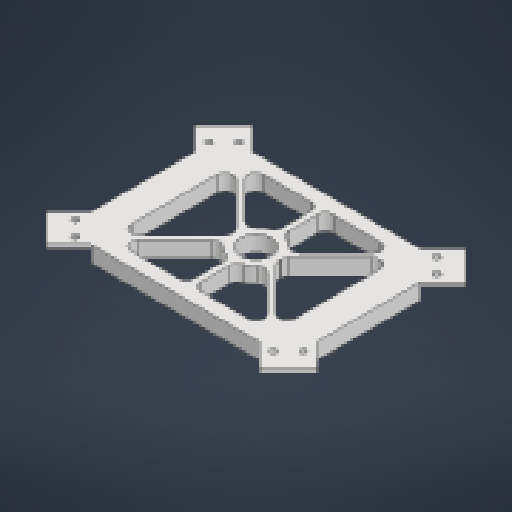
# Autodesk Inventor part: Base
Saved by Autodesk Inventor 2023 (Build 270158000, 158)
## iProperties
Created: 2023-01-21
Part Number: Base
Material: Generic
Document SubType Name: Modeling
Designer: Michael
Density: 1 g/cm^3
Appearance: Default
Author: Michael
Autodesk Inventor part; units mm, degrees
ref_plane "YZ Plane" through (0, 0, 0) normal (1, 0, 0) x (0, 1, 0)
ref_plane "XZ Plane" through (0, 0, 0) normal (0, 1, 0) x (-1, 0, 0)
ref_plane "XY Plane" through (0, 0, 0) normal (0, 0, 1) x (1, 0, 0)
sketch "Sketch1" plane through (0, 0, 0) normal (0, 1, 0) x (-1, 0, 0)
  line L0 (0, 0) -> (177.8, 0)
  line L1 (177.8, 0) -> (177.8, -127)
  line L2 (177.8, -127) -> (0, -127)
  line L3 (0, -127) -> (0, 0)
  line L4 (155.3506, 0) -> (177.8, -22.4519) projected
  line L5 (173.3121, 17.9595) -> (155.3506, 0) projected
  line L6 (195.7615, -4.4923) -> (173.3121, 17.9595) projected
  line L7 (177.8, -22.4519) -> (195.7615, -4.4923) projected
  line L8 (195.7615, -122.5077) -> (177.8, -104.5481) projected
  line L9 (173.3121, -144.9595) -> (195.7615, -122.5077) projected
  line L10 (155.3506, -127) -> (173.3121, -144.9595) projected
  line L11 (177.8, -104.5481) -> (155.3506, -127) projected
  line L12 (22.4494, 0) -> (4.4879, 17.9595) projected
  line L13 (0, -22.4519) -> (22.4494, 0) projected
  line L14 (4.4879, 17.9595) -> (-17.9615, -4.4923) projected
  line L15 (-17.9615, -4.4923) -> (0, -22.4519) projected
  line L16 (22.4494, -127) -> (0, -104.5481) projected
  line L17 (4.4879, -144.9595) -> (22.4494, -127) projected
  line L18 (0, -104.5481) -> (-17.9615, -122.5077) projected
  line L19 (-17.9615, -122.5077) -> (4.4879, -144.9595) projected
  circle A0 centre (178.6987, -10.7776) radius 2.4765
  circle A1 centre (167.025, 0.8974) radius 2.4765
  circle A2 centre (178.6987, -116.2224) radius 2.4765
  circle A3 centre (167.025, -127.8974) radius 2.4765
  circle A4 centre (10.775, -127.8974) radius 2.4765
  circle A5 centre (-0.8987, -116.2224) radius 2.4765
  circle A6 centre (-0.8987, -10.7776) radius 2.4765
  circle A7 centre (10.775, 0.8974) radius 2.4765
  dimension "d0" = 177.8
  dimension "d1" = 127
  constraints: 8 centre point, 8 end point, 2 parallel, 1 horizontal, 1 perpendicular, 16 other
  measures "d0" distance of L1.end L2.end
  measures "d1" distance of L0.end L1.end
extrude "Extrusion1" add sketch "Sketch1" along normal blind 12.7 contours L13 L3 A6 L0 A7 | L0 A7 L3 A6 L15 L14 L12 | L0 L4 L1 L11 L2 L16 L3 L13 | L5 L6 L7 L1 A0 L0 A1 | L0 A1 L1 A0 L4 | L16 L2 A4 L3 A5 | L3 A5 L2 A4 L17 L19 L18 | L8 L9 L10 L2 A3 L1 A2 | L1 A2 L2 A3 L11
sketch "Sketch6" plane through (0, 12.7, 0) normal (0, 1, 0) x (1, 0, 0)
  line L0 (-159.6708, 5.1549) -> (-18.3198, 5.1549)
  line L1 (-18.3198, 5.1549) -> (-18.3198, 121.9349)
  line L2 (-18.3198, 121.9349) -> (-159.6708, 121.9349)
  line L3 (-159.6708, 121.9349) -> (-159.6708, 5.1549)
  circle A0 centre (-88.9, 63.5) radius 12.2682
  line L4 (-24.5887, 14.5351) -> (-24.5887, 115.7894)
  line L5 (-24.5887, 115.7894) -> (-153.5245, 115.7894)
  line L6 (-153.5245, 115.7894) -> (-153.5245, 14.3771)
  line L7 (-153.5245, 112.7163) -> (-107.1207, 66.3124)
  line L8 (-153.5245, 112.7163) -> (-87.8995, 112.7163) construction
  line L9 (-150.4513, 115.7894) -> (-105.7361, 71.0742)
  line L10 (-153.5245, 14.3771) -> (-107.1207, 60.7809)
  line L11 (-150.4513, 11.3039) -> (-105.7651, 55.9901)
  line L12 (-24.5887, 112.7249) -> (-70.7001, 66.4653)
  line L13 (-27.4766, 115.7894) -> (-72.1058, 71.1763)
  line L14 (-24.4398, 14.3862) -> (-70.6864, 60.62)
  line L15 (-27.5134, 11.3039) -> (-72.0743, 55.8925)
  line L16 (-153.5245, 14.3771) -> (-107.1207, 60.7809)
  line L17 (-153.5245, 14.3771) -> (-153.5245, 63.5467)
  arc A1 (-70.6864, 60.62) -> (-70.7001, 66.4653) centre (-88.9, 63.5) ccw
  line L18 (-91.5188, 115.7894) -> (-91.519, 81.7746)
  line L19 (-86.6017, 115.7894) -> (-86.602, 81.8219)
  line L20 (-91.5188, 11.3039) -> (-91.519, 45.2251)
  line L21 (-86.6017, 11.3039) -> (-86.602, 45.1779)
  arc A2 (-86.602, 45.1779) -> (-72.0743, 55.8925) centre (-88.9, 63.5) ccw
  arc A3 (-72.1058, 71.1763) -> (-86.602, 81.8219) centre (-88.9, 63.5) ccw
  arc A4 (-91.519, 81.7746) -> (-105.7361, 71.0742) centre (-88.9, 63.5) ccw
  arc A5 (-107.1207, 66.3124) -> (-107.133, 60.7686) centre (-88.9, 63.5) ccw
  arc A6 (-105.7651, 55.9901) -> (-91.519, 45.2251) centre (-88.9, 63.5) ccw
  line L22 (-150.4513, 11.3039) -> (-91.5188, 11.3039)
  line L23 (-86.6017, 11.3039) -> (-27.5134, 11.3039)
  line L24 (-177.8, 104.5481) -> (-177.8, 22.4519) projected
  line L25 (0, 22.4519) -> (0, 104.5481) projected
  line L26 (0, 63.5) -> (-177.8, 63.5)
  line L27 (-22.4494, 127) -> (-155.3506, 127) projected
  line L28 (-88.9, 127) -> (-88.9, 0)
  point P0 (-203.2, 129.9481)
  point P1 (-203.2, 22.4519)
  point P2 (-180.7506, 0)
  point P3 (-22.4494, 0)
  point P4 (-25.3935, 140.9804)
  point P5 (-107.133, 60.7686)
  point P6 (-21.7778, 137.0134)
  point P7 (-177.8, 127)
  point P8 (-177.8, 0)
  dimension "d38" = 141.351
  dimension "d39" = 116.7799
  dimension "d42" = 24.5364
  dimension "d43" = 6.1463
  dimension "d45" = 45
  dimension "d46" = 45
  dimension "d47" = 3.0732
  dimension "d48" = 3.0732
  dimension "d54" = 4.917
  constraints: 60 end point, 12 point on circle, 9 point on line, 7 centre point, 5 parallel, 3 midpoint, 3 perpendicular, 2 collinear, 2 horizontal, 1 equal length, 1 vertical
  measures "d38" distance of L2.end L1.end
  measures "d39" distance of L1.end L0.end
  measures "d42" diameter of A0
  measures "d43" distance between parallel lines of L3 L6
  measures "d45" angle of L7 L8
  measures "d46" angle of L5 L9
  measures "d47" distance of L5.end L7.start
  measures "d48" distance of L9.start L5.end
  measures "d54" distance between parallel lines of L19 L18
extrude "Extrusion8" cut sketch "Sketch6" against normal blind 19.05 contours L28 L26 A0 | A0 L26 L28 | L26 A5 L10 L6 | L6 L7 A5 L26 | A0 L28 L26 | L26 L28 A0 | L26 A1 L12 L4 | L4 L14 A1 L26 | L5 L13 A3 L19 | L18 A4 L9 L5 | L11 A6 L20 L22 | L23 L21 A2 L15
fillet "Fillet1" radius 6.35 24 edges at (-70.7001, 6.35, -66.4653) (-70.6864, 6.35, -60.62) (-24.5887, 6.35, -14.5351) (-27.5134, 6.35, -11.3039) (-86.6017, 6.35, -11.3039) (-86.602, 6.35, -45.1779) (-72.0743, 6.35, -55.8925) (-86.6017, 6.35, -115.7894) (-86.602, 6.35, -81.8219) (-72.1058, 6.35, -71.1763) (-91.519, 6.35, -81.7746) (-105.7361, 6.35, -71.0742) (-150.4513, 6.35, -115.7894) (-91.5188, 6.35, -115.7894) (-153.5245, 6.35, -112.7163) (-107.1207, 6.35, -66.3124) (-107.133, 6.35, -60.7686) (-153.5245, 6.35, -14.3771) (-150.4513, 6.35, -11.3039) (-105.7651, 6.35, -55.9901) (-91.519, 6.35, -45.2251) (-91.5188, 6.35, -11.3039) (-27.4766, 6.35, -115.7894) (-24.5887, 6.35, -112.7249)
sketch "Sketch7" plane through (0, 0, 0) normal (0, -1, 0) x (1, 0, 0)
  arc A0 (-95.5736, -46.2868) -> (-102.0931, -50.5859) centre (-88.9, -63.5) ccw projected
  arc A1 (-111.1211, -50.6342) -> (-102.0931, -50.5859) centre (-106.631, -46.144) ccw projected
  line L0 (-111.1211, -50.6342) -> (-139.6112, -22.144) projected
  arc A2 (-135.1211, -11.3039) -> (-139.6112, -22.144) centre (-135.1211, -17.6539) ccw projected
  line L1 (-135.1211, -11.3039) -> (-97.8688, -11.3039) projected
  arc A3 (-91.5188, -17.6539) -> (-97.8688, -11.3039) centre (-97.8688, -17.6539) ccw projected
  line L2 (-91.5188, -17.6539) -> (-91.519, -40.3662) projected
  arc A4 (-95.5736, -46.2868) -> (-91.519, -40.3662) centre (-97.869, -40.3662) ccw projected
  circle A5 centre (-88.9, -63.5) radius 12.2682 projected
  line L3 (-153.5245, -97.386) -> (-153.5245, -29.7073) projected
  arc A6 (-142.6844, -25.2172) -> (-153.5245, -29.7073) centre (-147.1745, -29.7073) ccw projected
  line L4 (-142.6844, -25.2172) -> (-109.1944, -58.7071) projected
  arc A7 (-107.3351, -63.2748) -> (-109.1944, -58.7071) centre (-113.6846, -63.1972) ccw projected
  arc A8 (-107.3351, -63.2748) -> (-107.3341, -63.7937) centre (-88.9, -63.5) ccw projected
  arc A9 (-109.1932, -68.3849) -> (-107.3341, -63.7937) centre (-113.6833, -63.8948) ccw projected
  line L5 (-109.1932, -68.3849) -> (-142.6844, -101.8762) projected
  arc A10 (-153.5245, -97.386) -> (-142.6844, -101.8762) centre (-147.1745, -97.386) ccw projected
  line L6 (-24.5887, -29.8623) -> (-24.5887, -97.3598) projected
  arc A11 (-35.436, -101.8427) -> (-24.5887, -97.3598) centre (-30.9387, -97.3598) ccw projected
  line L7 (-35.436, -101.8427) -> (-68.6141, -68.558) projected
  arc A12 (-70.4651, -63.9278) -> (-68.6141, -68.558) centre (-64.1168, -64.0751) ccw projected
  arc A13 (-70.4651, -63.9278) -> (-70.4635, -63.1496) centre (-88.9, -63.5) ccw projected
  arc A14 (-68.6041, -58.5382) -> (-70.4635, -63.1496) centre (-64.1146, -63.029) ccw projected
  line L8 (-68.6041, -58.5382) -> (-35.4282, -25.3716) projected
  arc A15 (-24.5887, -29.8623) -> (-35.4282, -25.3716) centre (-30.9387, -29.8623) ccw projected
  line L9 (-42.8108, -115.7894) -> (-80.2518, -115.7894) projected
  arc A16 (-86.6018, -109.4395) -> (-80.2518, -115.7894) centre (-80.2518, -109.4394) ccw projected
  line L10 (-86.6018, -109.4395) -> (-86.6019, -86.7598) projected
  arc A17 (-82.4649, -80.8078) -> (-86.6019, -86.7598) centre (-80.2519, -86.7598) ccw projected
  arc A18 (-82.4649, -80.8078) -> (-75.7912, -76.505) centre (-88.9, -63.5) ccw projected
  arc A19 (-66.7939, -76.4863) -> (-75.7912, -76.505) centre (-71.2832, -80.9773) ccw projected
  line L11 (-66.7939, -76.4863) -> (-38.3215, -104.9485) projected
  arc A20 (-42.8108, -115.7894) -> (-38.3215, -104.9485) centre (-42.8108, -109.4394) ccw projected
  line L12 (-97.8688, -115.7894) -> (-135.1211, -115.7894) projected
  arc A21 (-139.6112, -104.9493) -> (-135.1211, -115.7894) centre (-135.1211, -109.4394) ccw projected
  line L13 (-139.6112, -104.9493) -> (-111.0747, -76.4128) projected
  arc A22 (-102.0585, -76.449) -> (-111.0747, -76.4128) centre (-106.5845, -80.9029) ccw projected
  arc A23 (-102.0585, -76.449) -> (-95.5735, -80.713) centre (-88.9, -63.5) ccw projected
  arc A24 (-91.519, -86.6335) -> (-95.5735, -80.713) centre (-97.869, -86.6336) ccw projected
  line L14 (-91.519, -86.6335) -> (-91.5188, -109.4394) projected
  arc A25 (-97.8688, -115.7894) -> (-91.5188, -109.4394) centre (-97.8688, -109.4394) ccw projected
  arc A26 (-75.7558, -50.5304) -> (-82.4649, -46.1919) centre (-88.9, -63.5) ccw projected
  arc A27 (-86.6019, -40.24) -> (-82.4649, -46.1919) centre (-80.2519, -40.24) ccw projected
  line L15 (-86.6019, -40.24) -> (-86.6018, -17.6539) projected
  arc A28 (-80.2518, -11.3039) -> (-86.6018, -17.6539) centre (-80.2518, -17.6539) ccw projected
  line L16 (-80.2518, -11.3039) -> (-42.8369, -11.3039) projected
  arc A29 (-38.3454, -22.1426) -> (-42.8369, -11.3039) centre (-42.8369, -17.6539) ccw projected
  line L17 (-38.3454, -22.1426) -> (-66.7442, -50.5591) projected
  arc A30 (-75.7558, -50.5304) -> (-66.7442, -50.5591) centre (-71.2358, -46.0704) ccw projected
  line L18 (-195.7615, -4.4923) -> (-173.3121, 17.9595) projected
  line L19 (-177.8, -22.4519) -> (-195.7615, -4.4923) projected
  line L20 (-177.8, -104.5481) -> (-177.8, -22.4519) projected
  line L21 (-195.7615, -122.5077) -> (-177.8, -104.5481) projected
  line L22 (-173.3121, -144.9595) -> (-195.7615, -122.5077) projected
  line L23 (-155.3506, -127) -> (-173.3121, -144.9595) projected
  line L24 (-22.4494, -127) -> (-155.3506, -127) projected
  line L25 (-4.4879, -144.9595) -> (-22.4494, -127) projected
  line L26 (17.9615, -122.5077) -> (-4.4879, -144.9595) projected
  line L27 (0, -104.5481) -> (17.9615, -122.5077) projected
  line L28 (0, -22.4519) -> (0, -104.5481) projected
  line L29 (17.9615, -4.4923) -> (0, -22.4519) projected
  line L30 (-4.4879, 17.9595) -> (17.9615, -4.4923) projected
  line L31 (-22.4494, 0) -> (-4.4879, 17.9595) projected
  line L32 (-155.3506, 0) -> (-22.4494, 0) projected
  line L33 (-173.3121, 17.9595) -> (-155.3506, 0) projected
  circle A31 centre (-178.6987, -116.2224) radius 2.2479 projected
  circle A32 centre (-167.025, -127.8974) radius 2.2479 projected
  circle A33 centre (0.8987, -116.2224) radius 2.2479 projected
  circle A34 centre (-10.775, -127.8974) radius 2.2479 projected
  circle A35 centre (-10.775, 0.8974) radius 2.2479 projected
  circle A36 centre (0.8987, -10.7776) radius 2.2479 projected
  line L34 (-155.3506, 0) -> (-22.4494, 0) projected
  line L35 (-22.4494, 0) -> (-4.4879, 17.9595) projected
  line L36 (-22.4494, 0) -> (-4.4879, 17.9595)
  line L37 (17.9615, -4.4923) -> (0, -22.4519) projected
  line L38 (-4.4879, 17.9595) -> (17.9615, -4.4923)
  line L39 (17.9615, -4.4923) -> (0, -22.4519)
  line L40 (0, -22.4519) -> (-22.4494, 0)
  line L41 (0, -22.4519) -> (0, -104.5481) projected
  line L42 (0, -63.5) -> (-177.8, -63.5)
  line L43 (-88.9, 0) -> (-88.9, -127)
  line L44 (-22.4494, -127) -> (-155.3506, -127) projected
  line L45 (17.9615, -122.5077) -> (0, -104.5481)
  line L46 (-4.4879, -144.9595) -> (17.9615, -122.5077)
  line L47 (-22.4494, -127) -> (-4.4879, -144.9595)
  circle A37 centre (-10.775, -127.8974) radius 2.2479
  circle A38 centre (0.8987, -116.2224) radius 2.2479
  line L48 (-22.4494, -127) -> (-4.4879, -144.9595)
  line L49 (-22.4494, -127) -> (-4.4879, -144.9595)
  line L50 (17.9615, -122.5077) -> (0, -104.5481)
  line L51 (-4.4879, -144.9595) -> (17.9615, -122.5077)
  line L52 (17.9615, -122.5077) -> (0, -104.5481)
  line L53 (0, -104.5481) -> (-22.4494, -127)
  line L54 (-173.3121, -144.9595) -> (-155.3506, -127)
  line L55 (-195.7615, -122.5077) -> (-173.3121, -144.9595)
  line L56 (-177.8, -104.5481) -> (-195.7615, -122.5077)
  line L57 (-195.7615, -4.4923) -> (-177.8, -22.4519)
  line L58 (-173.3121, 17.9595) -> (-195.7615, -4.4923)
  line L59 (-155.3506, 0) -> (-173.3121, 17.9595)
  line L60 (-177.8, -22.4519) -> (-155.3506, 0)
  line L61 (-177.8, -104.5481) -> (-155.3506, -127)
  point P0 (0, 0)
  point P1 (0, -127)
  constraints: 46 end point, 39 centre point, 4 midpoint, 3 symmetric about line, 2 collinear, 2 perpendicular, 3 other
extrude "Extrusion9" cut sketch "Sketch7" against normal blind 9.525 contours L60 L19 L18 L33 | L31 L30 L29 L40 | L53 L27 L26 L25 | L23 L22 L21 L61
body "Solid1"
